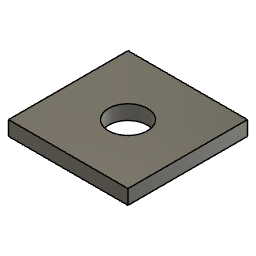
AE361-2 v1 (Autodesk Fusion 360 design; units mm, degrees)
Autodesk Fusion 360 part; units mm, degrees
sketch "Sketch1" plane through (0, 0, 0) normal (0, 1, 0) x (1, 0, 0)
  line L0 (0, 0) -> (-32.98, 0)
  line L1 (-32.98, 0) -> (-32.98, 32.98)
  line L2 (-32.98, 32.98) -> (0, 32.98)
  line L3 (0, 32.98) -> (0, 0)
  line L4 (-32.98, 16.49) -> (-32.98, 10)
  circle A0 centre (-16.49, 16.49) radius 5.37
  dimension "d1" = 32.98
  dimension "d2" = 32.98
  dimension "d3" = 6.49
  dimension "d5" = 10.74
  constraint horizontal L0
  constraint vertical L1
  constraint horizontal L2
  constraint vertical L3
  constraint coincident L0.start L3.end
  constraint midpoint L1 L4.start
  constraint coincident L1 L4.end
  measures "d1" distance of L0.start L0.end
  measures "d2" distance of L0.start L2.end
  measures "d3" distance of L4.start L4.end
  measures "d5" diameter of A0
extrude "Extrude1" add sketch "Sketch1" along normal blind 4
